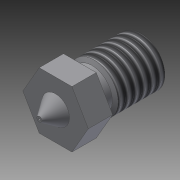
# Autodesk Inventor part: E3D_Nozzle
Saved by Autodesk Inventor 2014 (Build 180170000, 170)
## iProperties
Created: 2014-09-30
Part Number: E3D_Nozzle
Material: Generic
Document SubType Name: Modeling
Designer: ThatOtherGuy
Density: 1 g/cm^3
Appearance: Default
Author: ThatOtherGuy
Autodesk Inventor part; units mm, degrees
ref_plane "YZ Plane" through (0, 0, 0) normal (1, 0, 0) x (0, 1, 0)
ref_plane "XZ Plane" through (0, 0, 0) normal (0, 1, 0) x (-1, 0, 0)
ref_plane "XY Plane" through (0, 0, 0) normal (0, 0, 1) x (1, 0, 0)
sketch "Sketch1" plane through (0, 0, 0) normal (0, 0, 1) x (1, 0, 0)
  line L0 (0, 0) -> (0, 12.5)
  line L1 (0.125, 0) -> (0.315, 0)
  line L2 (0.315, 0) -> (1.7154, 2)
  line L3 (1.7154, 2) -> (3.1378, 2)
  line L4 (3.1378, 2) -> (3.1378, 5)
  line L5 (3.1378, 5) -> (2.5, 5)
  line L6 (2.5, 5) -> (2.5, 6.5)
  line L7 (2.5, 6.5) -> (3, 6.7211)
  line L8 (3, 6.7211) -> (3, 12.5)
  line L9 (3, 12.5) -> (1.5, 12.5)
  line L10 (1, 12) -> (1, 1.7)
  line L11 (1, 1.7) -> (0.5, 1.4789)
  line L12 (0.5, 1.4789) -> (0.5, 0.6658)
  line L13 (0.5, 0.6658) -> (0.125, 0.5)
  line L14 (0.125, 0.5) -> (0.125, 0)
  line L15 (1, 12) -> (1.5, 12.5)
  dimension "d0" = 0.25
  dimension "d1" = 0.63
  dimension "d2" = 1
  dimension "d3" = 0.5
  dimension "d4" = 10.8
  dimension "d5" = 2
  dimension "d6" = 12.5
  dimension "d7" = 125
  dimension "d8" = 10.5
  dimension "d9" = 7.5
  dimension "d10" = 6
  dimension "d11" = 6
  dimension "d12" = 5
  dimension "d13" = 45
  dimension "d14" = 3
  constraints: 32 end point, 8 parallel, 3 vertical, 2 perpendicular, 1 horizontal alignment
  measures "d0" diameter of L14 L0
  measures "d1" diameter of L1.end L0
  measures "d2" diameter of L12 L0
  measures "d3" distance of L1.start L13.end
  measures "d4" distance from line of L9 L10.end
  measures "d5" diameter of L10 L0
  measures "d6" distance between parallel lines of L9 L1
  measures "d7" angle of L3 L2
  measures "d8" distance between parallel lines of L9 L3
  measures "d9" distance between parallel lines of L9 L5
  measures "d10" distance from line of L9 L6.end
  measures "d11" diameter of L8 L0
  measures "d12" diameter of L6 L0
  measures "d13" angle of L9 L15
  measures "d14" diameter of L9.end L0
revolve "Revolution1" add sketch "Sketch1" angle 360 about axis through (0, 0, 0) along (0, 1, 0)
sketch "Sketch2" plane through (0, 2, 0) normal (0, -1, 0) x (1, 0, 0)
  circle A0 centre (0, 0) radius 3.1378 projected
  circle A1 centre (0, 0) radius 1.7154 projected
  line L0 (2.0207, 3.5) -> (4.0415, 0)
  line L1 (4.0415, 0) -> (2.0207, -3.5)
  line L2 (2.0207, -3.5) -> (-2.0207, -3.5)
  line L3 (-2.0207, -3.5) -> (-4.0415, 0)
  line L4 (-4.0415, 0) -> (-2.0207, 3.5)
  line L5 (-2.0207, 3.5) -> (2.0207, 3.5)
  dimension "d18" = 7
  constraints: 12 end point, 1 coincident, 1 horizontal, 13 other
  measures "d18" distance between parallel lines of L5 L2
extrude "Extrusion1" add sketch "Sketch2" against normal blind 3 contours L0 L1 L2 L3 L4 L5
thread "Thread1" size "M6x1" class "6g" standard "ANSI Metric M Profile" full length
body "Solid1"
